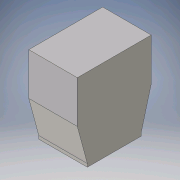
# Autodesk Inventor part: Upper_body_v2
Saved by Autodesk Inventor 2016 (Build 200138000, 138)
## iProperties
Created: 2018-11-02
Part Number: Upper_body_v2
Material: Generic
Document SubType Name: Modeling
Designer: attila
Density: 1 g/cm^3
Appearance: Default
Author: attila
Autodesk Inventor part; units mm, degrees
ref_plane "YZ Plane" through (0, 0, 0) normal (1, 0, 0) x (0, 1, 0)
ref_plane "XZ Plane" through (0, 0, 0) normal (0, 1, 0) x (-1, 0, 0)
sketch "Sketch1" plane through (0, 0, 0) normal (0, 1, 0) x (-1, 0, 0)
  line L0 (23, 25.5) -> (-23, 25.5)
  line L1 (-23, 25.5) -> (-23, -25.5)
  line L2 (-23, -25.5) -> (23, -25.5)
  line L3 (23, -25.5) -> (23, 25.5)
  point P0 (0, 0)
  point P1 (-23, 0)
  point P2 (23, 0)
  point P3 (0, 25.5)
  point P4 (0, -25.5)
  dimension "d0" = 46
  dimension "d1" = 51
  constraints: 8 end point, 4 midpoint, 2 horizontal alignment, 2 parallel, 1 horizontal, 1 perpendicular, 1 vertical alignment
  measures "d0" distance between parallel lines of L1 L3
  measures "d1" distance between parallel lines of L2 L0
extrude "Extrusion1" add sketch "Sketch1" along normal blind 3
sketch "Sketch2" plane through (0, 3, 0) normal (0, 1, 0) x (1, 0, 0)
  line L0 (-23, -25.5) -> (23, -25.5) projected
  line L1 (23, 25.5) -> (-23, 25.5) projected
  line L2 (-23, 25.5) -> (-23, -25.5) projected
  line L3 (23, -25.5) -> (23, 25.5) projected
  point P0 (0, 0)
  point P1 (-15, -17.5)
  point P2 (-15, 17.5)
  point P3 (15, -17.5)
  point P4 (15, 17.5)
  dimension "d4" = 8
  dimension "d5" = 8
  dimension "d6" = 8
  dimension "d7" = 8
  dimension "d8" = 8
  dimension "d9" = 8
  dimension "d10" = 8
  dimension "d11" = 8
  measures "d4" distance from line of L0 point (-15, -17.5)
  measures "d5" distance from line of L0 point (15, -17.5)
  measures "d6" distance from line of L1 point (15, 17.5)
  measures "d7" distance from line of L1 point (-15, 17.5)
  measures "d8" distance from line of L2 point (-15, -17.5)
  measures "d9" distance from line of L3 point (15, -17.5)
  measures "d10" distance from line of L3 point (15, 17.5)
  measures "d11" distance from line of L2 point (-15, 17.5)
hole "Hole1" at (-15, 3, 17.5) at (-15, 3, -17.5) at (15, 3, 17.5) at (15, 3, -17.5) direction (0, -1, 0) diameter 2 end through all
ref_plane "Work Plane1" through (23, 0, 25.5) normal (1, 0, 0) x (0, 0, -1)
sketch "Sketch3" plane through (23, 0, 25.5) normal (1, 0, 0) x (0, 0, -1)
  line L0 (25.5, 0) -> (25.5, 200)
  line L1 (60.5, 78.2142) -> (-9.5, 78.2142)
  line L2 (51, 3) -> (0, 3) projected
  line L3 (0, 3) -> (51, 3) projected
  line L4 (60.5, 78.2142) -> (60.5, 38.2142)
  line L5 (-9.5, 78.2142) -> (-9.5, 38.2142)
  line L6 (-9.5, 38.2142) -> (0, 3)
  line L7 (60.5, 38.2142) -> (51, 3)
  point P0 (25.5, 78.2142)
  point P1 (25.5, 3)
  point P2 (25.5, 3)
  dimension "d19" = 200
  dimension "d20" = 70
  dimension "d23" = 40
  dimension "d24" = 40
  constraints: 12 end point, 3 midpoint, 3 vertical, 1 coincident, 1 horizontal, 1 point on line
  measures "d19" distance of L0.start L0.end
  measures "d20" distance of L1.start L1.end
  measures "d23" distance of L1.start L4.end
  measures "d24" distance of L1.end L5.end
extrude "Extrusion3" add sketch "Sketch3" against normal blind 3
sketch "Sketch4" plane through (20, 0, 25.5) normal (-1, 0, 0) x (0, 0, 1)
  line L0 (-51, 3) -> (0, 3) projected
  line L1 (-60.5, 78.2142) -> (-60.5, 38.2142) projected
  line L2 (-51, 3) -> (-60.5, 38.2142)
  line L3 (9.5, 78.2142) -> (-60.5, 78.2142) projected
  line L4 (-60.5, 38.2142) -> (-60.5, 78.2142)
  line L5 (9.5, 38.2142) -> (9.5, 78.2142) projected
  line L6 (-60.5, 78.2142) -> (9.5, 78.2142)
  line L7 (0, 3) -> (9.5, 38.2142) projected
  line L8 (9.5, 78.2142) -> (9.5, 38.2142)
  line L9 (9.5, 38.2142) -> (0, 3)
  line L10 (-47.8927, 3) -> (-57.5, 38.6118)
  line L11 (-57.5, 38.6118) -> (-57.5, 75.2142)
  line L12 (-57.5, 75.2142) -> (6.5, 75.2142)
  line L13 (6.5, 75.2142) -> (6.5, 38.6118)
  line L14 (6.5, 38.6118) -> (-3.1073, 3)
  point P0 (-25.5, 0)
  dimension "d27" = 3
  dimension "d28" = 3
  dimension "d29" = 3
  dimension "d30" = 3
  dimension "d31" = 3
  constraints: 20 end point, 5 parallel, 3 perpendicular, 2 point on line, 1 collinear
  measures "d27" distance between parallel lines of L7 L14
  measures "d28" distance between parallel lines of L5 L13
  measures "d29" distance between parallel lines of L3 L12
  measures "d30" distance between parallel lines of L1 L11
  measures "d31" distance between parallel lines of L2 L10
extrude "Extrusion4" add sketch "Sketch4" along normal blind 43 contours L2 L1 L3 L5 L7 L0 L14 L13 L12 L11 L10
equation "\"d5\" = d10"
equation "\"d6\" = d4"
equation "\"d7\" = d8"
equation "\"d8\" = d4"
equation "\"d9\" = d10"
equation "\"d10\" = d6"
equation "\"d11\" = d7"
equation "\"d27\" = d28"
equation "\"d28\" = d29"
equation "\"d29\" = d30"
equation "\"d30\" = d31"
body "Solid1"
